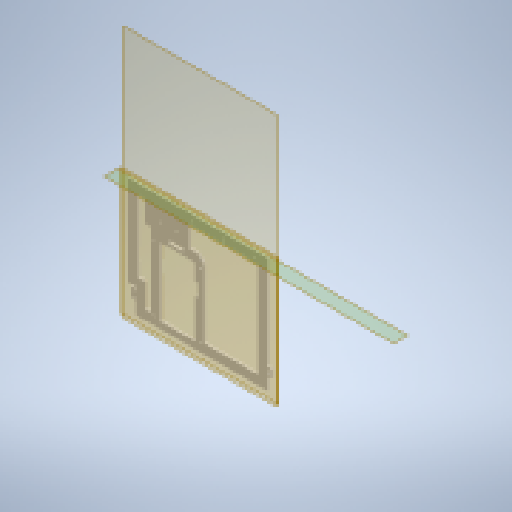
# Autodesk Inventor part: Pieza3
Saved by Autodesk Inventor 2023 (Build 270158000, 158)
## iProperties
Created: 2023-05-12
Part Number: Pieza3
Material: Genérico
Document SubType Name: Modeling
Designer: sergi
Density: 1 g/cm^3
Appearance: Valor por defecto
Author: sergi
Autodesk Inventor part; units mm, degrees
ref_plane "YZ Plane" through (0, 0, 0) normal (1, 0, 0) x (0, 1, 0)
ref_plane "XZ Plane" through (0, 0, 0) normal (0, 1, 0) x (-1, 0, 0)
ref_plane "XY Plane" through (0, 0, 0) normal (0, 0, 1) x (1, 0, 0)
ref_plane "Plano de trabajo1" through (0, 0, 0) normal (0, 0, 1) x (1, 0, 0)
sketch "Boceto1" plane through (0, 0, 0) normal (0, 0, 1) x (1, 0, 0)
  circle A0 centre (-100.65, -156.7) radius 1.65 projected
  circle A1 centre (-100.65, -148.3) radius 1.65 projected
  circle A2 centre (-100.65, 156.7) radius 1.65 projected
  circle A3 centre (-100.65, 148.3) radius 1.65 projected
  line L0 (-97.75, 145) -> (-105.25, 145) projected
  line L1 (-97.75, 142) -> (-97.75, 145) projected
  line L2 (-109, 142) -> (-97.75, 142) projected
  line L3 (-109, -142) -> (-109, 142) projected
  line L4 (-97.75, -142) -> (-109, -142) projected
  line L5 (-97.75, -145) -> (-97.75, -142) projected
  line L6 (-105.25, -145) -> (-97.75, -145) projected
  line L7 (-105.25, -160) -> (-105.25, -145) projected
  line L8 (-97.75, -160) -> (-105.25, -160) projected
  line L9 (-97.75, -180) -> (-97.75, -160) projected
  line L10 (109, -180) -> (-97.75, -180) projected
  line L11 (115.3, -160) -> (109, -160) projected
  line L12 (109, 146.9) -> (109, -146.9) projected
  line L13 (109, -146.9) -> (115.3, -146.9) projected
  line L14 (115.3, 146.9) -> (109, 146.9) projected
  line L15 (109, 180) -> (109, 160) projected
  line L16 (109, 160) -> (115.3, 160) projected
  line L17 (-97.75, 180) -> (109, 180) projected
  line L18 (-97.75, 160) -> (-97.75, 180) projected
  line L19 (-105.25, 160) -> (-97.75, 160) projected
  line L20 (-105.25, 145) -> (-105.25, 160) projected
  circle A4 centre (111.9, -156.3) radius 1.2 projected
  circle A5 centre (111.9, -150.6) radius 1.2 projected
  circle A6 centre (111.9, 156.3) radius 1.2 projected
  circle A7 centre (111.9, 150.6) radius 1.2 projected
  line L21 (115.3, -146.9) -> (115.3, -160) projected
  line L22 (115.3, 160) -> (115.3, 146.9) projected
  line L23 (109, -160) -> (109, -180) projected
  point P0 (0, 0)
extrude "Extrusión1" add sketch "Boceto1" along normal blind 3.9 contours A0 | A1 | A2 | A3 | L0 L20 L19 L18 L17 L15 L16 L22 L14 L12 L13 L21 L11 L23 L10 L9 L8 L7 L6 L5 L4 L3 L2 L1 | A4 | A5 | A6 | A7
sketch "Boceto3" plane through (0, 0, 0) normal (0, 0, -1) x (-1, 0, 0)
  line L0 (111, 180) -> (111, -185.2) projected
  line L1 (90.8, 170.8) -> (90.8, -176) projected
  line L2 (-99.7, -176) -> (-99.7, 170.8) projected
  line L3 (-117.3, 180) -> (-117.3, -185.2) projected
  line L4 (90.8, 170.8) -> (90.8, -176) projected
  line L5 (90.8, -176) -> (-99.7, -176) projected
  line L6 (-99.7, -176) -> (-99.7, 170.8) projected
  line L7 (-117.3, 180) -> (-117.3, -185.2) projected
  line L8 (109, -187.2) -> (-115.3, -187.2) projected
  line L9 (111, 180) -> (111, -185.2) projected
  circle A0 centre (-111.9, -150.6) radius 2.5 projected
  circle A1 centre (100.65, -148.3) radius 2.5 projected
  circle A2 centre (100.65, -156.7) radius 2.5 projected
  circle A3 centre (-111.9, -156.3) radius 2.5 projected
  arc A4 (-117.3, -185.2) -> (-115.3, -187.2) centre (-115.3, -185.2) ccw projected
  line L10 (109, -187.2) -> (-115.3, -187.2) projected
  arc A5 (109, -187.2) -> (111, -185.2) centre (109, -185.2) ccw projected
  circle A6 centre (-111.9, -150.6) radius 2.5 projected
  circle A7 centre (-111.9, -156.3) radius 2.5 projected
  arc A8 (-117.3, -185.2) -> (-115.3, -187.2) centre (-115.3, -185.2) ccw projected
  arc A9 (109, -187.2) -> (111, -185.2) centre (109, -185.2) ccw projected
  circle A10 centre (-111.9, 150.6) radius 2.5 projected
  circle A11 centre (100.65, -156.7) radius 2.5 projected
  circle A12 centre (100.65, 148.3) radius 2.5 projected
  circle A13 centre (100.65, 156.7) radius 2.5 projected
  circle A14 centre (100.65, -148.3) radius 2.5 projected
  circle A15 centre (-111.9, 156.3) radius 2.5 projected
  arc A16 (111, 180) -> (109, 182) centre (109, 180) ccw projected
  line L11 (109, 182) -> (-115.3, 182) projected
  arc A17 (-115.3, 182) -> (-117.3, 180) centre (-115.3, 180) ccw projected
  line L12 (-99.7, 170.8) -> (90.8, 170.8) projected
  line L13 (90.8, -176) -> (-99.7, -176) projected
  circle A18 centre (-111.9, 150.6) radius 2.5 projected
  circle A19 centre (100.65, 148.3) radius 2.5 projected
  circle A20 centre (100.65, 156.7) radius 2.5 projected
  circle A21 centre (-111.9, 156.3) radius 2.5 projected
  arc A22 (111, 180) -> (109, 182) centre (109, 180) ccw projected
  line L14 (109, 182) -> (-115.3, 182) projected
  arc A23 (-115.3, 182) -> (-117.3, 180) centre (-115.3, 180) ccw projected
  line L15 (-99.7, 170.8) -> (90.8, 170.8) projected
  point P0 (0, 0)
  point P1 (111, 0)
  point P2 (90.8, 0)
  point P3 (-99.7, 0)
  point P4 (-117.3, 0)
  constraints: 1 coincident
hole "Agujero1" at (-100.65, -148.3, 0) at (-100.65, -156.7, 0) at (111.9, -156.3, 0) at (111.9, -150.6, 0) at (-100.65, 156.7, 0) at (-100.65, 148.3, 0) at (111.9, 150.6, 0) at (111.9, 156.3, 0) direction (0, 0, 1) diameter 3 end through all
sketch "Boceto4" plane through (0, 0, 3.9) normal (0, 0, 1) x (1, 0, 0)
  line L0 (-59, -109.6) -> (-59, -139.7) projected
  line L1 (-59, -139.7) -> (-49.6, -139.7) projected
  line L2 (-49.6, -109.6) -> (-59, -109.6) projected
  line L3 (-59, -62.4) -> (-59, -169.5) projected
  line L4 (-3.9, -169.5) -> (-3.9, -62.4) projected
  line L5 (-3.9, -62.4) -> (-59, -62.4) projected
  line L6 (-59, -169.5) -> (-3.9, -169.5) projected
  line L7 (-49.6, -139.7) -> (-49.6, -109.6) projected
  point P0 (0, 0)
  point P1 (-3.9, -139.7)
  point P2 (-3.9, -109.6)
extrude "Extrusión2" cut sketch "Boceto4" against normal through all
sketch "Boceto5" plane through (0, 0, 3.9) normal (0, 0, 1) x (1, 0, 0)
  line L0 (-59, -62.4) -> (-3.9, -62.4) projected
  line L1 (-3.9, -62.4) -> (-3.9, -87.4)
  line L2 (-3.9, -109.6) -> (-3.9, -139.7) projected
  line L3 (-3.9, -87.4) -> (1.1, -87.4)
  line L4 (-3.9, -87.4) -> (1.1, -87.4) construction
  line L5 (1.1, -87.4) -> (1.1, -107.4)
  line L6 (1.1, -107.4) -> (-3.9, -107.4)
  line L7 (-3.9, -87.4) -> (-3.9, -107.4)
  point P0 (0, 0)
  point P1 (-3.9, -169.5)
  dimension "d11" = 25
  dimension "d12" = 5
  dimension "d13" = 0
  dimension "d14" = 20
  constraints: 12 end point, 4 perpendicular, 2 point on line, 1 collinear, 1 horizontal
  measures "d11" distance of L0.end L1.end
  measures "d12" distance of L1.end L3.end
  measures "d13" distance between parallel lines of L3 L4
  measures "d14" distance of L3.end L5.end
extrude "Extrusión3" cut sketch "Boceto5" against normal blind 4
sketch "Boceto6" plane through (0, 0, 0) normal (0, 0, -1) x (-1, 0, 0)
  line L0 (-1.1, -87.4) -> (-1.1, -107.4) projected
  line L1 (-1.1, -87.4) -> (-61.1, -87.4)
  line L2 (-61.1, -87.4) -> (-61.1, -107.4)
  line L3 (-61.1, -107.4) -> (-1.1, -107.4)
  line L4 (-1.1, -107.4) -> (-1.1, -87.4)
  point P0 (0, 0)
  dimension "d17" = 60
  constraints: 8 end point, 2 parallel, 1 horizontal, 1 perpendicular
  measures "d17" distance of L3.end L2.end
extrude "Extrusión4" cut sketch "Boceto6" against normal blind 1
sketch "Boceto7" plane through (0, 0, 0) normal (0, 0, -1) x (-1, 0, 0)
  line L0 (3.9, -109.6) -> (3.9, -139.7) projected
  line L1 (109, 142) -> (109, -142) projected
  line L2 (3.9, -87.4) -> (109, -87.4)
  line L3 (109, -87.4) -> (109, -107.4)
  line L4 (109, -107.4) -> (3.9, -107.4)
  line L5 (3.9, -107.4) -> (3.9, -87.4)
  point P0 (0, 0)
  point P1 (3.9, -107.4)
  point P2 (3.9, -107.4)
  dimension "d20" = 20
  constraints: 8 end point, 2 parallel, 1 horizontal, 1 perpendicular, 1 point on line
  measures "d20" distance of L2.end L3.end
extrude "Extrusión5" cut sketch "Boceto7" against normal blind 1
sketch "Boceto8" plane through (0, 0, 3.9) normal (0, 0, 1) x (1, 0, 0)
  line L0 (109, 180) -> (-97.75, 180) projected
  line L1 (0, 180) -> (0, -258.0429)
  line L2 (102.7, -146.9) -> (102.7, 146.9) projected
  line L3 (-109, 142) -> (-109, -142) projected
  line L4 (-109, 0) -> (102.7, 0)
  line L5 (-3.9, -87.4) -> (-3.9, -62.4) projected
  line L6 (-3.9, -62.4) -> (-59.3756, -62.4)
  line L7 (-59.3756, -62.4) -> (-59.3756, -169.7804)
  line L8 (-59.3756, -169.7804) -> (-3.9, -169.7804)
  line L9 (-3.9, -169.7804) -> (-3.9, -62.4)
  line L10 (-64.3756, -57.4) -> (1.1, -57.4)
  line L11 (1.1, -57.4) -> (1.1, -174.7804)
  line L12 (1.1, -174.7804) -> (-64.3756, -174.7804)
  line L13 (-64.3756, -174.7804) -> (-64.3756, -57.4)
  point P0 (0, 0)
  point P1 (102.7, 180)
  point P2 (0, -174.7804)
  point P3 (0, -57.4)
  dimension "d23" = 5
  constraints: 20 end point, 4 parallel, 3 perpendicular, 2 midpoint, 1 horizontal, 1 point on line, 3 other
  measures "d23" distance between parallel lines of L6 L10
extrude "Extrusión6" add sketch "Boceto8" along normal blind 16 contours L1 L12 L13 L10
sketch "Boceto9" plane through (-59.3756, -169.7804, 3.9) normal (1, 0, 0) x (0, 0, -1)
  line L0 (-0.9, 89.3804) -> (-0.9, 107.3804) projected
  line L1 (2.4, 107.3804) -> (-0.9, 107.3804) projected
  line L2 (2.4, 107.3804) -> (2.4, 0.2804) projected
  line L3 (2.4, 0.2804) -> (-0.9, 0.2804) projected
  line L4 (-0.9, 0.2804) -> (-0.9, 6.4804) projected
  line L5 (-0.9, 6.4804) -> (-12.4, 6.4804) projected
  line L6 (-12.4, 6.4804) -> (-12.4, 15.4804) projected
  line L7 (-12.4, 15.4804) -> (-0.9, 15.4804) projected
  line L8 (-0.9, 15.4804) -> (-0.9, 20.2804) projected
  line L9 (-0.9, 20.2804) -> (-10.2, 20.2804) projected
  line L10 (-10.2, 20.2804) -> (-10.2, 27.4804) projected
  line L11 (-10.2, 27.4804) -> (-0.9, 27.4804) projected
  line L12 (-0.9, 27.4804) -> (-0.9, 30.0804) projected
  line L13 (-0.9, 30.0804) -> (-13.95, 30.0804) projected
  line L14 (-13.95, 60.1804) -> (-13.95, 30.0804) projected
  line L15 (-13.95, 60.1804) -> (-0.9, 60.1804) projected
  line L16 (-0.9, 60.1804) -> (-0.9, 73.3804) projected
  line L17 (-0.9, 73.3804) -> (-7.6, 73.3804) projected
  line L18 (-7.6, 73.3804) -> (-7.6, 89.3804) projected
  line L19 (-7.6, 89.3804) -> (-0.9, 89.3804) projected
  line L20 (0, 107.3804) -> (0, 0) projected
  line L21 (0, 107.3804) -> (-16, 107.3804) projected
  line L22 (-16, 0) -> (-16, 107.3804) projected
  line L23 (0, 0) -> (-16, 0) projected
  line L24 (-0.9, 89.3804) -> (-0.9, 73.3804)
  line L25 (-0.9, 73.3804) -> (-0.9, 6.4804)
  point P0 (3.9, 169.7804)
  point P1 (-0.9, 15.4804)
  point P2 (-0.9, 20.2804)
  point P3 (-0.9, 27.4804)
  point P4 (-0.9, 30.0804)
  point P5 (-0.9, 60.1804)
  constraints: 4 end point, 1 collinear, 1 vertical
extrude "Extrusión7" cut sketch "Boceto9" against normal blind 15 contours L24 L17 L18 L19 | L25 L13 L14 L15 | L25 L9 L10 L11 | L5 L6 L7 L25
sketch "Boceto10" plane through (-59.3756, -169.7804, 3.9) normal (1, 0, 0) x (0, 0, -1)
  line L0 (-16, 0) -> (-16, 107.3804) projected
  line L1 (0, 107.3804) -> (-16, 107.3804) projected
  line L2 (-16, 0) -> (-13.95, 0)
  line L3 (-13.95, 0) -> (-13.95, 107.3804)
  line L4 (-13.95, 107.3804) -> (-16, 107.3804)
  line L5 (-16, 107.3804) -> (-16, 0)
  point P0 (3.9, 169.7804)
  dimension "d28" = 2.05
  constraints: 8 end point, 2 parallel, 1 horizontal, 1 perpendicular, 1 point on line
  measures "d28" distance of L4.end L3.end
extrude "Extrusión8" add sketch "Boceto10" along normal up to surface (55.4756 mm away)
sketch "Boceto11" plane through (-59.3756, -109.6, 17.85) normal (0, 0, -1) x (-1, 0, 0)
  line L0 (-14.4756, 41.2) -> (-36.6756, 41.2) projected
  line L1 (-36.6756, 41.2) -> (-36.6756, 47.2) projected
  line L2 (-14.4756, 47.2) -> (-14.4756, 41.2) projected
  line L3 (-14.4756, 47.2) -> (-36.6756, 47.2) projected
  line L4 (-0.3756, 29.2) -> (-12.3756, 29.2) projected
  line L5 (-12.3756, 13.2) -> (-12.3756, 29.2) projected
  line L6 (-0.3756, 13.2) -> (-12.3756, 13.2) projected
  line L7 (-0.3756, 13.2) -> (-0.3756, 29.2) projected
  line L8 (-0.3756, -44.7) -> (-15.3756, -44.7) projected
  line L9 (-0.3756, -53.7) -> (-15.3756, -53.7) projected
  line L10 (-15.3756, -53.7) -> (-15.3756, -44.7) projected
  line L11 (-0.3756, -39.9) -> (-26.3756, -39.9) projected
  line L12 (-0.3756, -32.7) -> (-26.3756, -32.7) projected
  line L13 (-26.3756, -39.9) -> (-26.3756, -32.7) projected
  line L14 (-9.7756, 0) -> (-9.7756, -30.1) projected
  line L15 (-9.7756, 0) -> (-0.3756, 0) projected
  line L16 (-0.3756, -32.7) -> (-26.3756, -32.7) projected
  line L17 (-0.3756, -32.7) -> (-26.3756, -32.7) projected
  line L18 (-0.3756, -30.1) -> (-9.7756, -30.1) projected
  arc A0 (-48.2506, 42.8) -> (-49.9006, 41.15) centre (-49.9006, 42.8) ccw projected
  circle A1 centre (-5.9506, 42.8) radius 1.65 projected
  circle A2 centre (-49.9006, -55.5) radius 1.65 projected
  circle A3 centre (-5.9506, -55.5) radius 1.65 projected
  line L19 (-55.4756, -60.1804) -> (-55.4756, 47.2) projected
  line L20 (-55.4756, 47.2) -> (-45.4756, 47.2)
  line L21 (-45.4756, 47.2) -> (-45.4756, 37.2)
  line L22 (-45.4756, 37.2) -> (-55.4756, 37.2)
  line L23 (-55.4756, 37.2) -> (-55.4756, 47.2)
  line L24 (-0.3756, 47.2) -> (-10.3756, 47.2)
  line L25 (-10.3756, 47.2) -> (-10.3756, 37.2)
  line L26 (-10.3756, 37.2) -> (-0.3756, 37.2)
  line L27 (-0.3756, 37.2) -> (-0.3756, 47.2)
  line L28 (0, -60.1804) -> (-55.4756, -60.1804) projected
  line L29 (-55.4756, -60.1804) -> (-45.4756, -60.1804)
  line L30 (-55.4756, -50.1804) -> (-55.4756, -60.1804)
  line L31 (-0.3756, -59.9) -> (-0.3756, 47.2) projected
  line L32 (-0.3756, -59.9) -> (-10.3756, -59.9)
  line L33 (-10.3756, -59.9) -> (-10.3756, -53.8)
  line L34 (-10.3756, -53.8) -> (-0.3756, -53.8)
  line L35 (-0.3756, -53.8) -> (-0.3756, -59.9)
  line L36 (-55.4756, -59.9) -> (-0.3756, -59.9) projected
  line L37 (-55.4756, -59.9) -> (-45.4756, -59.9)
  line L38 (-45.4756, -59.9) -> (-45.4756, -49.9)
  line L39 (-45.4756, -49.9) -> (-55.4756, -49.9)
  line L40 (-55.4756, -49.9) -> (-55.4756, -59.9)
  circle A4 centre (-49.9006, 42.8) radius 1.65
  point P0 (-59.3756, 109.6)
  point P1 (-0.3756, -53.8)
  dimension "d31" = 10
  dimension "d32" = 10
  dimension "d33" = 10
  dimension "d34" = 10
  dimension "d37" = 6.1
  dimension "d38" = 10
  dimension "d39" = 10
  constraints: 36 end point, 8 parallel, 5 horizontal, 4 perpendicular, 1 centre point, 1 coincident, 1 point on line, 1 other
  measures "d31" distance of L21.end L22.end
  measures "d32" distance of L20.end L21.end
  measures "d33" distance of L26.end L25.end
  measures "d34" distance of L25.end L24.end
  measures "d37" distance of L32.end L33.end
  measures "d38" distance of L39.end L38.end
  measures "d39" distance of L38.end L37.end
extrude "Extrusión9" add sketch "Boceto11" along normal blind 12.5 contours L19 L20 L21 L22 | L36 L19 L39 L38 | L31 L32 L33 L34 | L26 L25 L24 L27
sketch "Boceto12" plane through (-64.3756, -57.4, 3.9) normal (0, 1, 0) x (1, 0, 0)
  line L0 (41.6756, -0.9) -> (60.4756, -0.9) projected
  line L1 (60.4756, 2.4) -> (60.4756, -0.9) projected
  line L2 (60.4756, 2.4) -> (5.3756, 2.4) projected
  line L3 (5.3756, 2.4) -> (5.3756, -0.9) projected
  line L4 (5.3756, -0.9) -> (19.4756, -0.9) projected
  line L5 (19.4756, -0.9) -> (19.4756, -9.5) projected
  line L6 (19.4756, -9.5) -> (41.6756, -9.5) projected
  line L7 (41.6756, -9.5) -> (41.6756, -0.9) projected
  line L8 (19.4756, -0.9) -> (42.0812, -0.9)
  point P0 (64.3756, 3.9)
  constraints: 2 end point, 1 point on line
extrude "Extrusión10" cut sketch "Boceto12" against normal blind 12.5 contours L7 L6 L5 L8
sketch "Boceto13" plane through (0, 0, 3.9) normal (0, 0, 1) x (1, 0, 0)
  line L0 (-44.9, -57.4) -> (-22.7, -57.4) projected
  line L1 (-22.7, -57.4) -> (-44.9, -57.4)
  line L2 (-44.9, -57.4) -> (-44.9, -52.4)
  line L3 (-44.9, -52.4) -> (-22.7, -52.4)
  line L4 (-22.7, -52.4) -> (-22.7, -57.4)
  point P0 (0, 0)
  dimension "d44" = 5
  constraints: 8 end point, 2 parallel, 1 horizontal, 1 perpendicular
  measures "d44" distance of L1.end L2.end
extrude "Extrusión11" cut sketch "Boceto13" against normal blind 12.5
sketch "Boceto15" plane through (0, 0, 0) normal (0, 0, -1) x (-1, 0, 0)
  line L0 (22.7, 175.8) -> (22.7, -52.4) projected
  line L1 (44.9, -52.4) -> (44.9, 175.8) projected
  line L2 (44.9, 175.8) -> (22.7, 175.8) projected
  line L3 (18.5, 175.8) -> (44.9, 175.8) projected
  line L4 (-102.7, 175.8) -> (97.75, 175.8) projected
  line L5 (44.9, 157.7) -> (18.5, 157.7) projected
  line L6 (18.5, 157.7) -> (-90.5, 157.7) projected
  line L7 (-90.5, 180) -> (-90.5, 130) projected
  circle A0 centre (100.65, -156.7) radius 1.65 projected
  circle A1 centre (100.65, -148.3) radius 1.65 projected
  circle A2 centre (100.65, 156.7) radius 1.65 projected
  circle A3 centre (100.65, 148.3) radius 1.65 projected
  line L8 (97.75, 145) -> (105.25, 145) projected
  line L9 (105.25, 145) -> (105.25, 160) projected
  line L10 (105.25, 160) -> (97.75, 160) projected
  line L11 (97.75, 160) -> (97.75, 180) projected
  line L12 (97.75, 180) -> (-109, 180) projected
  line L13 (-109, 160) -> (-115.3, 160) projected
  line L14 (-109, -160) -> (-109, -180) projected
  line L15 (-115.3, 146.9) -> (-109, 146.9) projected
  line L16 (-109, -146.9) -> (-115.3, -146.9) projected
  line L17 (-109, 180) -> (-109, 160) projected
  line L18 (-115.3, -160) -> (-109, -160) projected
  line L19 (-109, -180) -> (97.75, -180) projected
  line L20 (97.75, -180) -> (97.75, -160) projected
  line L21 (97.75, -160) -> (105.25, -160) projected
  line L22 (105.25, -160) -> (105.25, -145) projected
  line L23 (105.25, -145) -> (97.75, -145) projected
  line L24 (97.75, -145) -> (97.75, -142) projected
  line L25 (97.75, -142) -> (109, -142) projected
  line L26 (109, -142) -> (109, 142) projected
  line L27 (109, 142) -> (97.75, 142) projected
  line L28 (97.75, 142) -> (97.75, 145) projected
  circle A4 centre (100.65, -156.7) radius 1.65 projected
  circle A5 centre (100.65, -148.3) radius 1.65 projected
  circle A6 centre (100.65, 156.7) radius 1.65 projected
  circle A7 centre (100.65, 148.3) radius 1.65 projected
  line L29 (97.75, 145) -> (105.25, 145) projected
  line L30 (105.25, 145) -> (105.25, 160) projected
  line L31 (105.25, 160) -> (97.75, 160) projected
  line L32 (97.75, 160) -> (97.75, 180) projected
  line L33 (97.75, 180) -> (-109, 180) projected
  line L34 (-109, 160) -> (-115.3, 160) projected
  line L35 (-109, -160) -> (-109, -180) projected
  line L36 (-115.3, 146.9) -> (-109, 146.9) projected
  line L37 (-109, -146.9) -> (-115.3, -146.9) projected
  line L38 (-109, 180) -> (-109, 160) projected
  line L39 (-115.3, -160) -> (-109, -160) projected
  line L40 (-109, -180) -> (97.75, -180) projected
  line L41 (97.75, -180) -> (97.75, -160) projected
  line L42 (97.75, -160) -> (105.25, -160) projected
  line L43 (105.25, -160) -> (105.25, -145) projected
  line L44 (105.25, -145) -> (97.75, -145) projected
  line L45 (97.75, -145) -> (97.75, -142) projected
  line L46 (97.75, -142) -> (109, -142) projected
  line L47 (109, -142) -> (109, 142) projected
  line L48 (109, 142) -> (97.75, 142) projected
  line L49 (97.75, 142) -> (97.75, 145) projected
  line L50 (44.9, -52.4) -> (44.9, -57.4) projected
  line L51 (22.7, -52.4) -> (44.9, -52.4) projected
  circle A8 centre (-111.9, -156.3) radius 1.2 projected
  circle A9 centre (-111.9, -150.6) radius 1.2 projected
  circle A10 centre (-111.9, 156.3) radius 1.2 projected
  circle A11 centre (-111.9, 150.6) radius 1.2 projected
  line L52 (-115.3, 160) -> (-115.3, 146.9) projected
  line L53 (-109, 146.9) -> (-109, -146.9) projected
  line L54 (-115.3, -146.9) -> (-115.3, -160) projected
  circle A12 centre (-111.9, -156.3) radius 1.2 projected
  circle A13 centre (-111.9, -150.6) radius 1.2 projected
  circle A14 centre (-111.9, 156.3) radius 1.2 projected
  circle A15 centre (-111.9, 150.6) radius 1.2 projected
  line L55 (-115.3, 160) -> (-115.3, 146.9) projected
  line L56 (-109, 146.9) -> (-109, -146.9) projected
  line L57 (-115.3, -146.9) -> (-115.3, -160) projected
  point P0 (0, 0)
  point P1 (-102.7, 180)
  point P2 (-102.7, 160)
  point P3 (-102.7, 146.9)
  point P4 (-102.7, -146.9)
  point P5 (-102.7, -160)
  point P6 (-102.7, -180)
  point P7 (-90.5, 175.8)
  point P8 (22.7, 157.7)
extrude "Extrusión13" cut sketch "Boceto15" against normal blind 2 contours L2 L1 L5 L0 | L0 L5 L6 L7 L4 L3 | L5 L1 L51 L0
sketch "Boceto16" plane through (0, 0, 2) normal (0, 0, -1) x (-1, 0, 0)
  line L0 (22.7, 157.7) -> (-90.5, 157.7) projected
  line L1 (-90.5, 157.7) -> (-81.3, 157.7)
  line L2 (-90.5, 157.7) -> (-81.3, 157.7) construction
  line L3 (-81.3, 157.7) -> (-81.3, 175.8645)
  line L4 (-90.5, 175.8) -> (44.9, 175.8) projected
  line L5 (-90.5, 175.8) -> (-90.5, 169.8)
  line L6 (-90.5, 157.7) -> (-90.5, 175.8) projected
  line L7 (-90.5, 169.8) -> (44.9, 169.8)
  line L8 (44.9, 175.8) -> (44.9, -52.4) projected
  line L9 (22.7, 157.7) -> (-90.5, 157.7) projected
  line L10 (-90.5, 157.7) -> (-90.5, 163.3)
  line L11 (-90.5, 163.3) -> (44.9, 163.3)
  line L12 (-81.3, 163.3) -> (-74.8, 163.3)
  line L13 (-74.8, 163.3) -> (-74.8, 169.8)
  line L14 (-74.8, 169.8) -> (-81.3, 169.8)
  line L15 (-81.3, 169.8) -> (-81.3, 163.3)
  line L16 (-90.5, 163.3) -> (-59.8, 163.3)
  line L17 (-59.8, 163.3) -> (-59.8, 169.8)
  line L18 (-59.8, 163.3) -> (-53.3, 163.3)
  line L19 (-53.3, 163.3) -> (-53.3, 169.8)
  line L20 (-53.3, 169.8) -> (-59.8, 169.8)
  line L21 (-59.8, 169.8) -> (-59.8, 163.3)
  line L22 (-90.5, 163.3) -> (-41.7, 163.3)
  line L23 (-41.7, 163.3) -> (-41.7, 169.8)
  line L24 (-41.7, 163.3) -> (-35.2, 163.3)
  line L25 (-35.2, 163.3) -> (-35.2, 169.8)
  line L26 (-35.2, 169.8) -> (-41.7, 169.8)
  line L27 (-41.7, 169.8) -> (-41.7, 163.3)
  line L28 (-90.5, 163.3) -> (-23.6, 163.3)
  line L29 (-90.5, 163.3) -> (-23.6, 163.3) construction
  line L30 (-23.6, 163.3) -> (-23.6, 169.8)
  line L31 (-23.6, 163.3) -> (-17.1, 163.3)
  line L32 (-17.1, 163.3) -> (-17.1, 169.8)
  line L33 (-17.1, 169.8) -> (-23.6, 169.8)
  line L34 (-23.6, 169.8) -> (-23.6, 163.3)
  line L35 (-90.5, 163.3) -> (-5.5, 163.3)
  line L36 (-90.5, 163.3) -> (-5.5, 163.3) construction
  line L37 (-5.5, 163.3) -> (1, 163.3)
  line L38 (1, 163.3) -> (1, 169.8)
  line L39 (1, 169.8) -> (-5.5, 169.8)
  line L40 (-5.5, 169.8) -> (-5.5, 163.3)
  line L41 (-90.5, 175.8) -> (44.9, 175.8) projected
  line L42 (-90.5, 175.8) -> (11.5, 175.8)
  line L43 (-90.5, 175.8) -> (11.5, 175.8) construction
  line L44 (11.5, 175.8) -> (11.5, 157.7)
  line L45 (11.5, 157.7) -> (19.5, 157.7)
  line L46 (19.5, 157.7) -> (19.5, 175.8)
  line L47 (19.5, 175.8) -> (11.5, 175.8)
  line L48 (11.5, 175.8) -> (11.5, 157.7)
  point P0 (0, 0)
  dimension "d58" = 9.2
  dimension "d59" = 0
  dimension "d60" = 6
  dimension "d61" = 5.6
  dimension "d62" = 6.5
  dimension "d63" = 30.7
  dimension "d64" = 6.5
  dimension "d65" = 6.5
  dimension "d66" = 48.8
  dimension "d67" = 6.5
  dimension "d68" = 6.5
  dimension "d69" = 66.9
  dimension "d70" = 0
  dimension "d71" = 90
  dimension "d72" = 6.5
  dimension "d73" = 6.5
  dimension "d74" = 85
  dimension "d75" = 0
  dimension "d76" = 6.5
  dimension "d77" = 6.5
  dimension "d80" = 102
  dimension "d81" = 0
  dimension "d82" = 8
  constraints: 86 end point, 13 point on line, 12 parallel, 11 perpendicular, 10 horizontal, 8 collinear, 1 vertical
  measures "d58" distance of L0.end L1.end
  measures "d59" distance between parallel lines of L1 L2
  measures "d60" distance of L4.start L5.end
  measures "d61" distance of L0.end L10.end
  measures "d62" distance of L14.end L13.end
  measures "d63" distance of L10.end L16.end
  measures "d64" distance of L20.end L19.end
  measures "d65" distance of L19.end L18.end
  measures "d66" distance of L10.end L22.end
  measures "d67" distance of L26.end L25.end
  measures "d68" distance of L25.end L24.end
  measures "d69" distance of L10.end L28.end
  measures "d70" distance between parallel lines of L28 L29
  measures "d71" angle of L30 L28
  measures "d72" distance of L33.end L32.end
  measures "d73" distance of L32.end L31.end
  measures "d74" distance of L10.end L35.end
  measures "d75" distance between parallel lines of L35 L36
  measures "d76" distance of L39.end L38.end
  measures "d77" distance of L38.end L37.end
  measures "d80" distance of L4.start L42.end
  measures "d81" distance between parallel lines of L43 L42
  measures "d82" distance of L47.end L46.end
extrude "Extrusión14" cut sketch "Boceto16" against normal through all contours L0 L44 L11 L46 | L11 L44 L7 L46 | L7 L44 L4 L46 | L3 L7 L13 L11 | L11 L40 L7 L38 | L17 L7 L19 L11 | L11 L30 L7 L32 | L23 L7 L25 L11
fillet "Empalme1" radius 5 5 edges at (0, -116.0902, 19.9) (-32.1878, -57.4, 19.9) (0, -57.4, 11.9) (-32.1878, -174.7804, 19.9) (0, -174.7804, 11.9)
sketch "Boceto17" plane through (-59.3756, -109.6, 17.85) normal (0, 0, -1) x (-1, 0, 0)
  line L0 (-0.3756, -32.7) -> (-26.3756, -32.7) projected
  line L1 (-26.3756, -39.9) -> (-26.3756, -32.7) projected
  line L2 (-0.3756, -39.9) -> (-26.3756, -39.9) projected
  line L3 (-26.3756, -32.7) -> (-15.3756, -32.7)
  line L4 (-15.3756, -32.7) -> (-15.3756, -39.9)
  line L5 (-15.3756, -39.9) -> (-26.3756, -39.9)
  line L6 (-26.3756, -39.9) -> (-26.3756, -32.7)
  point P0 (-59.3756, 109.6)
  point P1 (-15.3756, -32.7)
  dimension "d84" = 11
  constraints: 8 end point, 2 parallel, 1 horizontal, 1 perpendicular, 1 point on line
  measures "d84" distance of L4.end L5.end
extrude "Extrusión15" cut sketch "Boceto17" against normal blind 16
ref_plane "Plano de trabajo2" through (-97.75, 0, 0) normal (0, -1, 0) x (1, 0, 0)
fillet "Empalme3" radius 5 4 edges at (-13.9, -72.4, 11.6) (-49, -72.4, 11.6) (-13.9, -159.5, 11.6) (-49, -163.4, 11.6)
sketch "Boceto22" plane through (0, 0, 0) normal (0, 0, -1) x (-1, 0, 0)
  circle A0 centre (59, -35) radius 1.5 projected
  circle A1 centre (59, 35) radius 1.5 projected
  circle A2 centre (34, -35) radius 1.5 projected
  circle A3 centre (34, 35) radius 1.5 projected
  arc A4 (29, -35) -> (34, -40) centre (34, -35) ccw projected
  line L0 (29, -35) -> (29, 35) projected
  arc A5 (34, 40) -> (29, 35) centre (34, 35) ccw projected
  line L1 (34, 40) -> (59, 40) projected
  arc A6 (64, 35) -> (59, 40) centre (59, 35) ccw projected
  line L2 (64, 35) -> (64, -35) projected
  arc A7 (59, -40) -> (64, -35) centre (59, -35) ccw projected
  line L3 (59, -40) -> (34, -40) projected
  arc A8 (55.6519, 33) -> (59, 31.1) centre (59, 35) ccw projected
  line L4 (37.3481, 33) -> (55.6519, 33) projected
  arc A9 (34, 31.1) -> (37.3481, 33) centre (34, 35) ccw projected
  line L5 (34, 31.1) -> (34, 22) projected
  line L6 (59, 22) -> (34, 22) projected
  line L7 (59, 22) -> (59, 31.1) projected
  line L8 (59, -31.1) -> (59, -22) projected
  line L9 (34, -22) -> (59, -22) projected
  line L10 (34, -22) -> (34, -31.1) projected
  arc A10 (37.3481, -33) -> (34, -31.1) centre (34, -35) ccw projected
  line L11 (55.6519, -33) -> (37.3481, -33) projected
  arc A11 (59, -31.1) -> (55.6519, -33) centre (59, -35) ccw projected
  point P0 (0, 0)
hole "Agujero5" at (-59, 35, 0) at (-59, -35, 0) direction (0, 0, 1) diameter 3.2 end through all countersink diameter 6 countersink angle 90
sketch "Boceto24" plane through (0, 0, 2) normal (0, 0, -1) x (-1, 0, 0)
  circle A0 centre (59, -35) radius 1.5 projected
  circle A1 centre (59, 35) radius 1.5 projected
  circle A2 centre (34, -35) radius 1.5 projected
  circle A3 centre (34, 35) radius 1.5 projected
  arc A4 (29, -35) -> (34, -40) centre (34, -35) ccw projected
  line L0 (29, -35) -> (29, 35) projected
  arc A5 (34, 40) -> (29, 35) centre (34, 35) ccw projected
  line L1 (34, 40) -> (59, 40) projected
  arc A6 (64, 35) -> (59, 40) centre (59, 35) ccw projected
  line L2 (64, 35) -> (64, -35) projected
  arc A7 (59, -40) -> (64, -35) centre (59, -35) ccw projected
  line L3 (59, -40) -> (34, -40) projected
  arc A8 (55.6519, 33) -> (59, 31.1) centre (59, 35) ccw projected
  line L4 (37.3481, 33) -> (55.6519, 33) projected
  arc A9 (34, 31.1) -> (37.3481, 33) centre (34, 35) ccw projected
  line L5 (34, 31.1) -> (34, 22) projected
  line L6 (59, 22) -> (34, 22) projected
  line L7 (59, 22) -> (59, 31.1) projected
  line L8 (59, -31.1) -> (59, -22) projected
  line L9 (34, -22) -> (59, -22) projected
  line L10 (34, -22) -> (34, -31.1) projected
  arc A10 (37.3481, -33) -> (34, -31.1) centre (34, -35) ccw projected
  line L11 (55.6519, -33) -> (37.3481, -33) projected
  arc A11 (59, -31.1) -> (55.6519, -33) centre (59, -35) ccw projected
  point P0 (0, 0)
hole "Agujero6" at (-34, -35, 2) at (-34, 35, 2) direction (0, 0, 1) diameter 3.2 end through all
sketch "Boceto25" plane through (0, 0, 3.9) normal (0, 0, 1) x (1, 0, 0)
  circle A0 centre (-34, -35) radius 1.6 projected
  circle A1 centre (-34, 35) radius 1.6 projected
  circle A2 centre (-59, 35) radius 1.6 projected
  circle A3 centre (-59, -35) radius 1.6 projected
  line L0 (23.6, 169.8) -> (23.6, 163.3) projected
  line L1 (23.6, 163.3) -> (17.1, 163.3) projected
  line L2 (17.1, 163.3) -> (17.1, 169.8) projected
  line L3 (17.1, 169.8) -> (23.6, 169.8) projected
  line L4 (81.3, 169.8) -> (81.3, 163.3) projected
  line L5 (81.3, 163.3) -> (74.8, 163.3) projected
  line L6 (74.8, 163.3) -> (74.8, 169.8) projected
  line L7 (74.8, 169.8) -> (81.3, 169.8) projected
  line L8 (-1, 163.3) -> (-1, 169.8) projected
  line L9 (-1, 169.8) -> (5.5, 169.8) projected
  line L10 (5.5, 169.8) -> (5.5, 163.3) projected
  line L11 (5.5, 163.3) -> (-1, 163.3) projected
  line L12 (41.7, 169.8) -> (41.7, 163.3) projected
  line L13 (41.7, 163.3) -> (35.2, 163.3) projected
  line L14 (35.2, 163.3) -> (35.2, 169.8) projected
  line L15 (35.2, 169.8) -> (41.7, 169.8) projected
  line L16 (59.8, 169.8) -> (59.8, 163.3) projected
  line L17 (59.8, 163.3) -> (53.3, 163.3) projected
  line L18 (53.3, 163.3) -> (53.3, 169.8) projected
  line L19 (53.3, 169.8) -> (59.8, 169.8) projected
  line L20 (-11.5, 175.8) -> (-11.5, 157.7) projected
  line L21 (-11.5, 157.7) -> (-19.5, 157.7) projected
  line L22 (-19.5, 157.7) -> (-19.5, 175.8) projected
  line L23 (-19.5, 175.8) -> (-11.5, 175.8) projected
  line L24 (-22.7, -52.4) -> (-22.7, -57.4) projected
  line L25 (-22.7, -57.4) -> (-5, -57.4) projected
  arc A4 (0, -62.4) -> (-5, -57.4) centre (-5, -62.4) ccw projected
  line L26 (0, -62.4) -> (0, -87.4) projected
  line L27 (0, -87.4) -> (1.1, -87.4) projected
  line L28 (1.1, -87.4) -> (1.1, -107.4) projected
  line L29 (1.1, -107.4) -> (0, -107.4) projected
  line L30 (0, -107.4) -> (0, -169.7804) projected
  arc A5 (-5, -174.7804) -> (0, -169.7804) centre (-5, -169.7804) ccw projected
  line L31 (-5, -174.7804) -> (-64.3756, -174.7804) projected
  line L32 (-64.3756, -174.7804) -> (-64.3756, -57.4) projected
  line L33 (-64.3756, -57.4) -> (-44.9, -57.4) projected
  line L34 (-44.9, -57.4) -> (-44.9, -52.4) projected
  line L35 (-44.9, -52.4) -> (-22.7, -52.4) projected
  circle A6 centre (111.9, 150.6) radius 1.5 projected
  circle A7 centre (-100.65, 156.7) radius 1.5 projected
  circle A8 centre (111.9, -156.3) radius 1.5 projected
  circle A9 centre (-100.65, -148.3) radius 1.5 projected
  circle A10 centre (-100.65, -156.7) radius 1.5 projected
  circle A11 centre (111.9, -150.6) radius 1.5 projected
  circle A12 centre (-100.65, 148.3) radius 1.5 projected
  circle A13 centre (111.9, 156.3) radius 1.5 projected
  line L36 (-97.75, 142) -> (-109, 142) projected
  line L37 (-109, 142) -> (-109, -142) projected
  line L38 (-109, -142) -> (-97.75, -142) projected
  line L39 (-97.75, -142) -> (-97.75, -145) projected
  line L40 (-97.75, -145) -> (-105.25, -145) projected
  line L41 (-105.25, -145) -> (-105.25, -160) projected
  line L42 (-105.25, -160) -> (-97.75, -160) projected
  line L43 (-97.75, -160) -> (-97.75, -180) projected
  line L44 (-97.75, -180) -> (109, -180) projected
  line L45 (109, -180) -> (109, -160) projected
  line L46 (109, -160) -> (115.3, -160) projected
  line L47 (115.3, -160) -> (115.3, -146.9) projected
  line L48 (115.3, -146.9) -> (109, -146.9) projected
  line L49 (109, -146.9) -> (109, 146.9) projected
  line L50 (109, 146.9) -> (115.3, 146.9) projected
  line L51 (115.3, 146.9) -> (115.3, 160) projected
  line L52 (115.3, 160) -> (109, 160) projected
  line L53 (109, 160) -> (109, 180) projected
  line L54 (109, 180) -> (-97.75, 180) projected
  line L55 (-97.75, 180) -> (-97.75, 160) projected
  line L56 (-97.75, 160) -> (-105.25, 160) projected
  line L57 (-105.25, 160) -> (-105.25, 145) projected
  line L58 (-105.25, 145) -> (-97.75, 145) projected
  line L59 (-97.75, 145) -> (-97.75, 142) projected
  line L60 (109, -180) -> (109, 180)
  line L61 (-22.7, -52.4) -> (-22.7, 157.7) projected
  line L62 (-22.7, 157.7) -> (-19.5, 157.7) projected
  line L63 (-19.5, 175.8) -> (-44.9, 175.8) projected
  line L64 (-97.75, -180) -> (109, -180)
  line L65 (9, -165) -> (94, -165)
  line L66 (-22.7, -57.4) -> (-22.7, 157.7) projected
  line L67 (-14.7, 142.7) -> (94, 142.7)
  line L68 (-44.9, -57.4) -> (-64.3756, -57.4)
  line L69 (-44.9, -57.4) -> (-22.7, -57.4) projected
  line L70 (-97.75, -180) -> (-97.75, -142)
  line L71 (-97.75, 142) -> (-97.75, 180)
  line L72 (9, -165) -> (9, -116.4)
  line L73 (9, -116.4) -> (9, -62.4)
  arc A14 (9, -62.4) -> (-5, -48.4) centre (-5, -62.4) ccw
  line L74 (-5, -48.4) -> (-14.7, -48.4)
  line L75 (-94, 127) -> (-82.75, 127)
  line L76 (-82.75, 127) -> (-82.75, 145)
  line L77 (-82.75, 145) -> (-82.75, 165)
  line L78 (94, -145) -> (94, -165)
  line L79 (-82.75, -165) -> (-82.75, -160)
  line L80 (-82.75, -160) -> (-82.75, -127)
  line L81 (-82.75, -127) -> (-94, -127)
  line L82 (9, -78.4) -> (9, -62.4)
  arc A15 (9, -62.4) -> (-5, -48.4) centre (-5, -62.4) ccw
  line L83 (-5, -48.4) -> (-14.7, -48.4)
  line L84 (-82.75, 48.4) -> (-53.9, 48.4)
  line L85 (-82.75, 142.7) -> (-82.75, 127)
  line L86 (-73.3756, -48.4) -> (-73.3756, -165)
  line L87 (-82.75, -48.4) -> (-73.3756, -48.4)
  line L88 (-44.9, 175.8) -> (-44.9, -52.4) projected
  line L89 (-82.75, 48.4) -> (-82.75, 15)
  line L90 (-82.75, -15) -> (-82.75, -48.4)
  line L91 (-14.7, 15) -> (94, 15)
  line L92 (-14.7, -15) -> (94, -15)
  line L93 (-82.75, -15) -> (-94, -15)
  line L94 (-94, -127) -> (-94, -15)
  line L95 (-94, 15) -> (-94, 127)
  line L96 (-82.75, -165) -> (-73.3756, -165)
  line L97 (-73.3756, -165) -> (-82.75, -165)
  line L98 (94, -165) -> (9, -165)
  line L99 (9, -165) -> (94, -165)
  line L100 (-82.75, 15) -> (-94, 15)
  line L101 (-14.7, -57.4) -> (-14.7, -15)
  line L102 (-14.7, 15) -> (-14.7, 142.7)
  line L103 (94, -15) -> (94, -145)
  line L104 (94, -165) -> (94, -15)
  line L105 (94, -165) -> (94, -15)
  line L106 (94, -165) -> (94, -15)
  line L107 (94, 15) -> (94, 142.7)
  line L108 (94, 15) -> (94, 142.7)
  line L109 (94, 15) -> (94, 142.7)
  line L110 (94, 142.7) -> (94, 15)
  line L111 (-53.9, 48.4) -> (-53.9, 165)
  line L112 (-82.75, 165) -> (-53.9, 165)
  point P0 (0, 0)
  dimension "d143" = 9
  constraints: 95 end point, 5 perpendicular, 5 vertical, 4 point on circle, 3 point on line, 2 centre point, 2 horizontal, 2 parallel, 1 collinear, 5 other
  measures "d143" distance between parallel lines of L26 L73
extrude "Extrusión17" cut sketch "Boceto25" against normal blind 10 contours L101 L92 L103 L78 L65 L72 L73 A14 L74 | L67 L107 L91 L102 | L75 L76 L77 L112 L111 L84 L89 L100 L95 | L79 L80 L81 L94 L93 L90 L87 L86 L96
sketch "Boceto26" plane through (0, 0, 3.9) normal (0, 0, 1) x (1, 0, 0)
  line L0 (0, -107.4) -> (0, -169.7804) projected
  line L1 (0, -169.7804) -> (5, -169.7804)
  line L2 (5, -169.7804) -> (5, -162.7804)
  line L3 (5, -162.7804) -> (0, -162.7804)
  circle A0 centre (5, -166.2804) radius 2
  circle A1 centre (5, -166.2804) radius 3.5
  arc A2 (0, -62.4) -> (-5, -57.4) centre (-5, -62.4) ccw projected
  line L4 (0, -62.4) -> (5, -62.4)
  line L5 (5, -62.4) -> (5, -69.4)
  line L6 (5, -69.4) -> (0, -69.4)
  line L7 (0, -62.4) -> (0, -87.4) projected
  circle A3 centre (5, -65.9) radius 3.5
  circle A4 centre (5, -65.9) radius 2
  line L8 (-64.3756, -62.4) -> (-5, -62.4) projected
  line L9 (-64.3756, -62.4) -> (-69.3756, -62.4)
  line L10 (-69.3756, -62.4) -> (-69.3756, -69.4)
  line L11 (-69.3756, -69.4) -> (-63.3756, -69.4)
  line L12 (-64.3756, -62.4) -> (-64.3756, -169.7804) projected
  line L13 (-64.3756, -169.7804) -> (-69.3756, -169.7804)
  line L14 (-69.3756, -169.7804) -> (-69.3756, -163.3004)
  line L15 (-69.3756, -163.3004) -> (-64.3756, -163.3004)
  line L16 (-64.3756, -163.3004) -> (-64.3756, -169.7804)
  circle A5 centre (-69.3756, -65.9) radius 3.5
  circle A6 centre (-69.3756, -65.9) radius 2
  circle A7 centre (-69.3756, -166.5404) radius 2
  circle A8 centre (-69.3756, -166.5404) radius 3.24
  line L17 (-64.3756, -163.3) -> (-64.3756, -154.3) projected
  point P0 (0, 0)
  point P1 (-69.3756, -163.3004)
  point P2 (5, -169.7804)
  point P3 (5, -162.7804)
  point P4 (-64.3756, -69.4)
  dimension "d155" = 5
  dimension "d156" = 7
  dimension "d157" = 4
  dimension "d158" = 5
  dimension "d159" = 7
  dimension "d160" = 4
  dimension "d161" = 5
  dimension "d162" = 7
  dimension "d163" = 5
  dimension "d164" = 6.48
  dimension "d165" = 4
  dimension "d166" = 4
  constraints: 26 end point, 7 perpendicular, 5 centre point, 4 coincident, 4 horizontal, 4 midpoint, 2 parallel, 2 point on line, 1 tangent, 10 other
  measures "d155" distance of L0.end L1.end
  measures "d156" distance of L1.end L2.end
  measures "d157" diameter of A0
  measures "d158" distance of L4.start L4.end
  measures "d159" distance of L4.end L5.end
  measures "d160" diameter of A4
  measures "d161" distance of L8.start L9.end
  measures "d162" distance of L9.end L10.end
  measures "d163" distance of L14.end L15.end
  measures "d164" distance of L13.end L14.end
  measures "d165" diameter of A6
  measures "d166" diameter of A7
extrude "Extrusión18" add sketch "Boceto26" along normal blind 3.5 contours L3 A1 L1 L0 | A1 L2 A0 | L2 A0 A1 | L4 A3 L6 L7 | A3 L5 A4 | L5 A4 A3 | L12 L11 A5 L9 | L12 L13 A8 L15 | A5 L10 A6 | L10 A6 A5 | A8 L14 A7 | L14 A7 A8
fillet "Empalme4" radius 5 7 edges at (0, -169.7804, 5.65) (0, -162.7804, 5.65) (0, -62.4, 5.65) (0, -69.4, 5.65) (-64.3756, -169.7804, 5.65) (-64.3756, -62.4, 5.65) (-64.3756, -69.4, 5.65)
sketch "Boceto27" plane through (0, 0, 0) normal (0, 0, -1) x (-1, 0, 0)
  circle A0 centre (-111.9, -156.3) radius 1.2 projected
  circle A1 centre (-111.9, -150.6) radius 1.2 projected
  circle A2 centre (-111.9, 156.3) radius 1.2 projected
  circle A3 centre (-111.9, 150.6) radius 1.2 projected
  circle A4 centre (100.65, -156.7) radius 1.65 projected
  circle A5 centre (100.65, -148.3) radius 1.65 projected
  circle A6 centre (100.65, 156.7) radius 1.65 projected
  circle A7 centre (100.65, 148.3) radius 1.65 projected
  line L0 (-115.3, -160) -> (-109, -160) projected
  line L1 (-109, -160) -> (-109, -180) projected
  line L2 (-109, -180) -> (97.75, -180) projected
  line L3 (97.75, -180) -> (97.75, -160) projected
  line L4 (97.75, -160) -> (105.25, -160) projected
  line L5 (105.25, -160) -> (105.25, -145) projected
  line L6 (105.25, -145) -> (97.75, -145) projected
  line L7 (97.75, -145) -> (97.75, -142) projected
  line L8 (97.75, -142) -> (109, -142) projected
  line L9 (109, -142) -> (109, 142) projected
  line L10 (109, 142) -> (97.75, 142) projected
  line L11 (97.75, 142) -> (97.75, 145) projected
  line L12 (97.75, 145) -> (105.25, 145) projected
  line L13 (105.25, 145) -> (105.25, 160) projected
  line L14 (105.25, 160) -> (97.75, 160) projected
  line L15 (97.75, 160) -> (97.75, 180) projected
  line L16 (97.75, 180) -> (-109, 180) projected
  line L17 (-109, 180) -> (-109, 160) projected
  line L18 (-109, 160) -> (-115.3, 160) projected
  line L19 (-115.3, 160) -> (-115.3, 146.9) projected
  line L20 (-115.3, 146.9) -> (-109, 146.9) projected
  line L21 (-109, 146.9) -> (-109, -146.9) projected
  line L22 (-109, -146.9) -> (-115.3, -146.9) projected
  line L23 (-115.3, -146.9) -> (-115.3, -160) projected
  line L24 (64.3756, -57.4) -> (64.3756, -74.4) projected
  arc A8 (64.3756, -57.4) -> (69.3756, -62.4) centre (69.3756, -57.4) ccw projected
  arc A9 (69.3756, -69.4) -> (69.3756, -62.4) centre (69.3756, -65.9) ccw projected
  arc A10 (69.3756, -69.4) -> (64.3756, -74.4) centre (69.3756, -74.4) ccw projected
  circle A11 centre (69.3756, -65.9) radius 2 projected
  line L25 (64.3756, -163.3004) -> (64.3756, -174.7804) projected
  line L26 (64.3756, -163.3004) -> (69.3756, -163.3004) projected
  arc A12 (69.3756, -169.7804) -> (69.3756, -163.3004) centre (69.3756, -166.5404) ccw projected
  arc A13 (69.3756, -169.7804) -> (64.3756, -174.7804) centre (69.3756, -174.7804) ccw projected
  circle A14 centre (69.3756, -166.5404) radius 2 projected
  line L27 (0, -169.7804) -> (0, -157.7804) projected
  arc A15 (0, -169.7804) -> (0.6699, -172.2804) centre (5, -169.7804) ccw projected
  arc A16 (0.6699, -172.2804) -> (-3.6603, -169.7804) centre (-3.6603, -174.7804) ccw projected
  line L28 (-3.6603, -169.7804) -> (-5, -169.7804) projected
  arc A17 (-5, -162.7804) -> (-5, -169.7804) centre (-5, -166.2804) ccw projected
  arc A18 (-5, -162.7804) -> (0, -157.7804) centre (-5, -157.7804) ccw projected
  circle A19 centre (-5, -166.2804) radius 2 projected
  line L29 (0, -74.4) -> (0, -62.4) projected
  arc A20 (0, -74.4) -> (-5, -69.4) centre (-5, -74.4) ccw projected
  arc A21 (-5, -62.4) -> (-5, -69.4) centre (-5, -65.9) ccw projected
  line L30 (-5, -62.4) -> (-3.6603, -62.4) projected
  arc A22 (-3.6603, -62.4) -> (0.6699, -59.9) centre (-3.6603, -57.4) ccw projected
  arc A23 (0.6699, -59.9) -> (0, -62.4) centre (5, -62.4) ccw projected
  circle A24 centre (-5, -65.9) radius 2 projected
  point P0 (0, 0)
hole "Agujero7" at (-69.3756, -65.9, 0) at (-69.3756, -166.5404, 0) at (5, -166.2804, 0) at (5, -65.9, 0) direction (0, 0, 1) diameter 3 depth 3.9 countersink diameter 6 countersink angle 90
sketch "Boceto29" plane through (0, 0, 0) normal (0, 0, -1) x (-1, 0, 0)
  line L0 (14.7, 15) -> (-94, 15) projected
  line L1 (-94, -15) -> (14.7, -15)
  line L2 (14.7, -15) -> (14.7, 15)
  line L3 (14.7, 15) -> (-94, 15)
  line L4 (-94, 15) -> (-94, -15)
  line L5 (8.7, -9) -> (-88, -9)
  line L6 (-88, -9) -> (-88, 9)
  line L7 (-88, 9) -> (8.7, 9)
  line L8 (8.7, 9) -> (8.7, -9)
  circle A0 centre (8.7, -9) radius 1.5
  circle A1 centre (-88, -9) radius 1.5
  circle A2 centre (-88, 9) radius 1.5
  circle A3 centre (8.7, 9) radius 1.5
  circle A4 centre (-39.65, 9) radius 1.5
  circle A5 centre (-39.65, -9) radius 1.5
  point P0 (0, 0)
  dimension "d183" = 6
  dimension "d184" = 3
  dimension "d185" = 3
  dimension "d186" = 3
  dimension "d187" = 3
  dimension "d188" = 3
  dimension "d189" = 3
  constraints: 16 end point, 6 centre point, 4 coincident, 4 parallel, 2 midpoint, 2 perpendicular, 1 horizontal, 3 other
  measures "d183" distance between parallel lines of L1 L5
  measures "d184" diameter of A0
  measures "d185" diameter of A1
  measures "d186" diameter of A2
  measures "d187" diameter of A3
  measures "d188" diameter of A4
  measures "d189" diameter of A5
hole "Agujero8" at (-8.7, -9, 0) at (-8.7, 9, 0) at (39.65, 9, 0) at (39.65, -9, 0) at (88, -9, 0) at (88, 9, 0) direction (0, 0, 1) diameter 3 depth 3.9 countersink diameter 6 countersink angle 90
split "Dividir6" plane through (0, 0, 0) removes the side toward (0, 1, 0)
ref_plane "Plano de trabajo4" through (0, 0, 3.9) normal (0, 0, 1) x (1, 0, 0)
split "Dividir7" plane through (0, 0, 3.9) removes the side toward (0, 0, 1)
